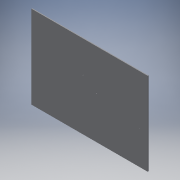
# Autodesk Inventor part: endplate
Saved by Autodesk Inventor 2018.2 (Build 222227000, 227)
## iProperties
Created: 2018-02-23
Part Number: endplate
Material: 一般
Document SubType Name: Modeling
Designer: ku_sk
Density: 1 g/cm^3
Appearance: 既定
Author: ku_sk
Autodesk Inventor part; units mm, degrees
ref_plane "YZ Plane" through (0, 0, 0) normal (1, 0, 0) x (0, 1, 0)
ref_plane "XZ Plane" through (0, 0, 0) normal (0, 1, 0) x (-1, 0, 0)
ref_plane "XY Plane" through (0, 0, 0) normal (0, 0, 1) x (1, 0, 0)
sketch "スケッチ1" plane through (0, 0, 0) normal (0, 1, 0) x (-1, 0, 0)
  line L0 (-250, 250) -> (250, 250)
  line L1 (250, 250) -> (250, -250)
  line L2 (250, -250) -> (-250, -250)
  line L3 (-250, -250) -> (-250, 250)
  line L4 (-250, 250) -> (250, -250) construction
  line L5 (250, 250) -> (-250, -250) construction
  point P0 (0, 0)
  dimension "d0" = 500
  dimension "d1" = 500
  constraints: 12 end point, 2 midpoint, 2 parallel, 1 horizontal, 1 perpendicular
  measures "d0" distance of L0.start L0.end
  measures "d1" distance of L2.end L0.start
extrude "押し出し1" add sketch "スケッチ1" along normal mid plane 5
sketch "スケッチ3" plane through (0, -2.5, 0) normal (0, -1, 0) x (1, 0, 0)
  circle A0 centre (-30, 105) radius 2.5
  line L0 (250, -250) -> (250, 250) projected
  line L1 (-250, -250) -> (250, -250) projected
  circle A1 centre (-110, 160) radius 2.5
  circle A2 centre (230, 50) radius 2.5
  point P0 (0, 0)
  dimension "d10" = 5
  dimension "d15" = 5
  dimension "d16" = 300
  dimension "d17" = 20
  dimension "d18" = 5
  dimension "d24" = 55
  dimension "d25" = 260
  dimension "d26" = 340
  dimension "d27" = 110
  constraints: 3 centre point
  measures "d10" diameter of A0
  measures "d15" diameter of A1
  measures "d16" distance from line of L1 A2.centre
  measures "d17" distance from line of L0 A2.centre
  measures "d18" diameter of A2
  measures "d24" vertical distance of A0.centre A2.centre
  measures "d25" horizontal distance of A0.centre A2.centre
  measures "d26" horizontal distance of A1.centre A2.centre
  measures "d27" vertical distance of A2.centre A1.centre
extrude "押し出し4" cut sketch "スケッチ3" against normal through all
sketch "スケッチ5" plane through (0, -2.5, 0) normal (0, -1, 0) x (1, 0, 0)
  line L0 (250, 250) -> (-250, 250) projected
  line L1 (-250, 250) -> (-250, -250) projected
  line L2 (-250, -250) -> (250, -250) projected
  line L3 (250, -250) -> (250, 250) projected
  line L4 (-250, 250) -> (250, 250) projected
  line L5 (-150, 250) -> (250, 110)
  line L6 (250, 250) -> (250, -250) projected
  line L7 (-250, -250) -> (-250, 250) projected
  line L8 (-250, 100) -> (-100, -50)
  line L9 (-100, -50) -> (85.1514, -50)
  line L10 (85.1514, -50) -> (250, 10)
  point P0 (0, 0)
  dimension "d30" = 100
  dimension "d32" = 100
  dimension "d33" = 150
  dimension "d34" = 300
  dimension "d35" = 45
  dimension "d36" = 20
  dimension "d37" = 60
  constraints: 8 end point, 4 point on line, 1 horizontal
  measures "d30" distance of L10.end L5.end
  measures "d32" distance from line of L5.start L1
  measures "d33" distance from line of L0 L8.start
  measures "d34" distance between parallel lines of L0 L9
  measures "d35" angle of L9 L8
  measures "d36" angle of L9 L10
  measures "d37" distance from line of L9 L10.end
extrude "押し出し5" cut sketch "スケッチ5" against normal through all contours L3 L5 L0 | L3 L2 L1 L8 L9 L10
